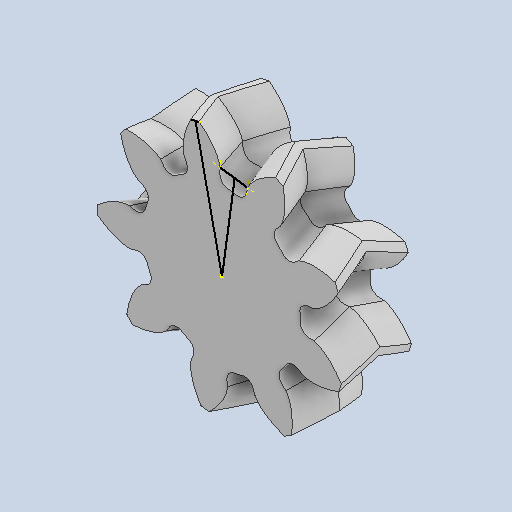
# Autodesk Inventor part: SmallGearV7
Saved by Autodesk Inventor 2022 (Build 260153070, 153G)
## iProperties
Created: 2022-01-26
Part Number: SmallGearV7
Material: Generic
Document SubType Name: Modeling
Designer: a laptop
Density: 1 g/cm^3
Appearance: Default
Author: a laptop
Autodesk Inventor part; units mm, degrees
ref_plane "YZ Plane" through (0, 0, 0) normal (1, 0, 0) x (0, 1, 0)
ref_plane "XZ Plane" through (0, 0, 0) normal (0, 1, 0) x (-1, 0, 0)
ref_plane "XY Plane" through (0, 0, 0) normal (0, 0, 1) x (1, 0, 0)
sketch "Sketch1" plane through (0, 0, 0) normal (0, 0, 1) x (1, 0, 0)
  spline S0 degree 3 poles (-1.652933, 5.062213) (-1.596511, 5.028864) (-1.483659, 4.962162) (-1.32306, 4.848488) (-1.169171, 4.726031) (-1.02434, 4.59287) (-0.890188, 4.448964) (-0.769085, 4.293781) (-0.682999, 4.154093) (-0.625197, 4.036211) (-0.604945, 3.973841) (-0.594822, 3.942664) knots 0 0 0 0 0.12501294 0.25004151 0.37505906 0.50007142 0.62507639 0.75006761 0.87502761 0.93752969 1 1 1 1
  spline S1 degree 3 poles (-0.594822, 3.942664) (-0.594963, 3.901251) (-0.595246, 3.818443) (-0.578672, 3.694762) (-0.538925, 3.576497) (-0.482521, 3.487588) (-0.420398, 3.432516) (-0.368189, 3.398204) (-0.309612, 3.376511) (-0.187134, 3.352172) (0, 3.385873) (0.187134, 3.352172) (0.309612, 3.376511) (0.368189, 3.398204) (0.420398, 3.432516) (0.482521, 3.487588) (0.538925, 3.576497) (0.578672, 3.694762) (0.595246, 3.818443) (0.594963, 3.901251) (0.594822, 3.942664) knots 0 0 0 0 0.06252795 0.12503102 0.187529 0.24989599 0.2811821 0.31241976 0.3436915 0.374932 0.5 0.625068 0.6563085 0.68758024 0.7188179 0.75010401 0.812471 0.87496898 0.93747205 1 1 1 1
  spline S2 degree 3 poles (0.594822, 3.942664) (0.604945, 3.973841) (0.625197, 4.036211) (0.682999, 4.154093) (0.769085, 4.293781) (0.890188, 4.448964) (1.02434, 4.59287) (1.169171, 4.726031) (1.32306, 4.848488) (1.483659, 4.962162) (1.596511, 5.028864) (1.652933, 5.062213) knots 0 0 0 0 0.06247031 0.12497239 0.24993239 0.37492361 0.49992858 0.62494094 0.74995849 0.87498706 1 1 1 1
  circle A0 centre (0, 0) radius 3.370893 construction
  circle A1 centre (0, 0) radius 3.961719 construction
  circle A2 centre (0, 0) radius 4.07048 construction
  circle A3 centre (0, 0) radius 5.32524
  point P0 (-1.485112, 4.959896)
  point P1 (-1.324174, 4.847021)
  point P2 (-1.170677, 4.724244)
  point P3 (-1.026115, 4.591075)
  point P4 (-0.892355, 4.447076)
  point P5 (-0.772041, 4.291693)
  point P6 (-0.669476, 4.124122)
  point P7 (-0.627353, 4.035339)
  point P8 (-0.592412, 3.818513)
  point P9 (-0.574804, 3.695644)
  point P10 (-0.534234, 3.578348)
  point P11 (-0.465637, 3.475224)
  point P12 (-0.419447, 3.433671)
  point P13 (-0.367143, 3.400315)
  point P14 (-0.309153, 3.378094)
  point P15 (-0.248322, 3.365904)
  point P16 (0, 3.370893)
  point P17 (0.248322, 3.365904)
  point P18 (0.309153, 3.378094)
  point P19 (0.367143, 3.400315)
  point P20 (0.419447, 3.433671)
  point P21 (0.465637, 3.475224)
  point P22 (0.534234, 3.578348)
  point P23 (0.574804, 3.695644)
  point P24 (0.592412, 3.818513)
  point P25 (0.627353, 4.035339)
  point P26 (0.669476, 4.124122)
  point P27 (0.772041, 4.291693)
  point P28 (0.892355, 4.447076)
  point P29 (1.026115, 4.591075)
  point P30 (1.170677, 4.724244)
  point P31 (1.324174, 4.847021)
  point P32 (1.485112, 4.959896)
  constraints: 4 centre point, 2 point on circle, 81 other
sketch "Sketch1 outline for Extrusion1" plane through (0, 0, 0) normal (0, 0, 1) x (1, 0, 0)
  circle A0 centre (0, 0) radius 5.32524
extrude "Extrusion1" add sketch "Sketch1 outline for Extrusion1" against normal blind 1.5
sketch "Sketch1 outline for Coil1" plane through (0, 0, 0) normal (0, 0, 1) x (1, 0, 0)
  arc A0 (1.652933, 5.062213) -> (-1.652933, 5.062213) centre (0, 0) ccw
  spline S0 degree 3 poles (0.594822, 3.942664) (0.604945, 3.973841) (0.625197, 4.036211) (0.682999, 4.154093) (0.769085, 4.293781) (0.890188, 4.448964) (1.02434, 4.59287) (1.169171, 4.726031) (1.32306, 4.848488) (1.483659, 4.962162) (1.596511, 5.028864) (1.652933, 5.062213) knots 0 0 0 0 0.06247031 0.12497239 0.24993239 0.37492361 0.49992858 0.62494094 0.74995849 0.87498706 1 1 1 1
  spline S1 degree 3 poles (-0.594822, 3.942664) (-0.594963, 3.901251) (-0.595246, 3.818443) (-0.578672, 3.694762) (-0.538925, 3.576497) (-0.482521, 3.487588) (-0.420398, 3.432516) (-0.368189, 3.398204) (-0.309612, 3.376511) (-0.187134, 3.352172) (0, 3.385873) (0.187134, 3.352172) (0.309612, 3.376511) (0.368189, 3.398204) (0.420398, 3.432516) (0.482521, 3.487588) (0.538925, 3.576497) (0.578672, 3.694762) (0.595246, 3.818443) (0.594963, 3.901251) (0.594822, 3.942664) knots 0 0 0 0 0.06252795 0.12503102 0.187529 0.24989599 0.2811821 0.31241976 0.3436915 0.374932 0.5 0.625068 0.6563085 0.68758024 0.7188179 0.75010401 0.812471 0.87496898 0.93747205 1 1 1 1
  spline S2 degree 3 poles (-1.652933, 5.062213) (-1.596511, 5.028864) (-1.483659, 4.962162) (-1.32306, 4.848488) (-1.169171, 4.726031) (-1.02434, 4.59287) (-0.890188, 4.448964) (-0.769085, 4.293781) (-0.682999, 4.154093) (-0.625197, 4.036211) (-0.604945, 3.973841) (-0.594822, 3.942664) knots 0 0 0 0 0.12501294 0.25004151 0.37505906 0.50007142 0.62507639 0.75006761 0.87502761 0.93752969 1 1 1 1
coil "Coil1" sketch "Sketch1 outline for Coil1" operation cut axis through (0, 0, -10) along (0, 0, -1) pitch 70.268674 turns 0.021347 hand right
pattern_circular "Circular Pattern1" count 9 over 360 about axis through (0, 0, -10) along (0, 0, 1) of "Coil1"
mirror "Mirror1" about plane through (0, 4.590599, 0) normal (0, 0, 1) of "Extrusion1", "Coil1", "Circular Pattern1"
sketch "Sketch3" plane through (0.487597, 3.613318, 1.5) normal (0, 0, 1) x (0.9905564, -0.137106, 0)
  arc A0 (-1.657792, 1.410492) -> (-1.992149, 1.287501) centre (0.012415, -3.646048) ccw
  line L0 (-1.992149, 1.287501) -> (-1.657792, 1.410492)
  line L1 (-1.824971, 1.348996) -> (0.012415, -3.646048)
  line L2 (-0.611786, 0.298624) -> (0.593772, 0.298624)
  line L3 (0.012415, 0.298624) -> (0.012415, -3.646048)
  point P0 (-0.595865, 0.294562)
  constraints: 8 end point, 2 perpendicular, 1 horizontal, 1 midpoint, 1 point on line
equation "\"d0\" = FaceWidth"
equation "\"Module\" = 0.85"
equation "\"PressureAngle\" = 12.5deg"
equation "\"UnitProfileClearance\" = 0.25"
equation "\"UnitRoundRadius\" = 0.3025"
equation "\"HeadDiameter\" = 10.65048"
equation "\"RootDiameter\" = 6.74179"
equation "\"BaseDiameter\" = 7.92344"
equation "\"PitchDiameter\" = 8.14096"
equation "\"FaceWidth\" = 1.5"
equation "\"HelixAngle\" = 20deg"
equation "\"UnitCorrection\" = 0.481312"
equation "\"UnitAddendumModification\" = 0.005123"
equation "\"CircularPitch\" = 2.84173"
equation "\"UnitBacklashShift\" = -0.054356"
equation "\"TotalToolShift\" = 0.36291"
equation "\"IsInternal\" = 0"
body "Solid1"
